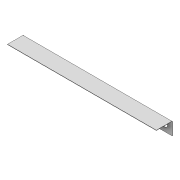
# Autodesk Inventor part: perfil_fijacion
Saved by Autodesk Inventor 2021 (Build 250183000, 183)
## iProperties
Created: 2021-06-13
Part Number: perfil_fijacion
Material: Genérico
Document SubType Name: Chapa
Designer: carlo
Density: 1 g/cm^3
Sheet Metal Rule: Por defecto_mm
Appearance: Valor por defecto
Author: carlo
Autodesk Inventor part; units mm, degrees
ref_plane "YZ Plane" through (0, 0, 0) normal (1, 0, 0) x (0, 1, 0)
ref_plane "XZ Plane" through (0, 0, 0) normal (0, 1, 0) x (-1, 0, 0)
ref_plane "XY Plane" through (0, 0, 0) normal (0, 0, 1) x (1, 0, 0)
sketch "Boceto1" plane through (0, 0, 0) normal (0, 0, 1) x (1, 0, 0)
  line L0 (0, 0) -> (460, 0)
  line L1 (460, 0) -> (460, 40)
  line L2 (460, 40) -> (0, 40)
  line L3 (0, 40) -> (0, 0)
  dimension "d0" = 460
  dimension "d1" = 40
  measures "d0" distance of L2.end L1.end
  measures "d1" distance of L1.end L0.end
extrude "Placa1" add sketch "Boceto1" along normal blind 1
sketch "Boceto2" plane through (0, 39, 0) normal (0, 1, 0) x (-1, 0, 0)
  line L0 (-460, 0) -> (0, 0)
  line L1 (0, 0) -> (0, 50)
  line L2 (0, 50) -> (-460, 50)
  line L3 (-460, 50) -> (-460, 0)
  constraints: 6 end point, 1 horizontal, 1 perpendicular, 1 vertical
edge flange "Pestaña1" height 50 angle 90 thickness 1 bend radius 1 thickness toward (0, 1, 0) relief tear relief width 1 relief depth 0.5 edges at (230, 40, 1) wall of the first edge with corners at (460, 39, 0) (0, 39, 0) (0, 39, 50) (460, 39, 50)
bend "Doblez1"
corner "Esquina1"
sketch "Boceto3" plane through (0, 0, 1) normal (0, 0, 1) x (1, 0, 0)
  circle A0 centre (23.3423, 20.935) radius 8.73
  circle A1 centre (436.5993, 20.935) radius 8.73
  line L0 (0, 0) -> (0, 38) projected
  line L1 (460, 40) -> (0, 40) projected
  dimension "d13" = 413.257
  dimension "d14" = 23.3423
  dimension "d15" = 17.46
  dimension "d16" = 17.46
  dimension "d17" = 19.065
  constraints: 2 centre point
  measures "d13" distance of A0.centre A1.centre
  measures "d14" distance from line of L0 A0.centre
  measures "d15" diameter of A1
  measures "d16" diameter of A0
  measures "d17" distance from line of L1 A0.centre
extrude "Extrusión1" cut sketch "Boceto3" against normal blind 10
equation "\"d16\" = d15"
equation "\"d2\" = Grosor"
equation "\"d3\" = Anchura_desahogo_plegado"
equation "\"d4\" = Profundidad_desahogo_plegado"
equation "\"d5\" = Remanente_mínimo"
equation "\"d6\" = Radiodetransición"
equation "\"d9\" = Radio_pliegue"
equation "\"d10\" = Tamaño_destalonado"
equation "\"d11\" = TamañoSeparación"
equation "\"d12\" = Tamaño_de_radio_de_Jacobi"
equation "\"Radio_pliegue\" = Grosor"
equation "\"Anchura_desahogo_plegado\" = Grosor"
equation "\"Profundidad_desahogo_plegado\" = 0.5 * Grosor"
equation "\"Tamaño_destalonado\" = 4 * Grosor"
equation "\"Remanente_mínimo\" = 2 * Grosor"
equation "\"Radiodetransición\" = Radio_pliegue"
equation "\"Tamaño_de_radio_de_Jacobi\" = Radio_pliegue"
equation "\"TamañoSeparación\" = Grosor"
equation "\"Grosor\" = 1"
